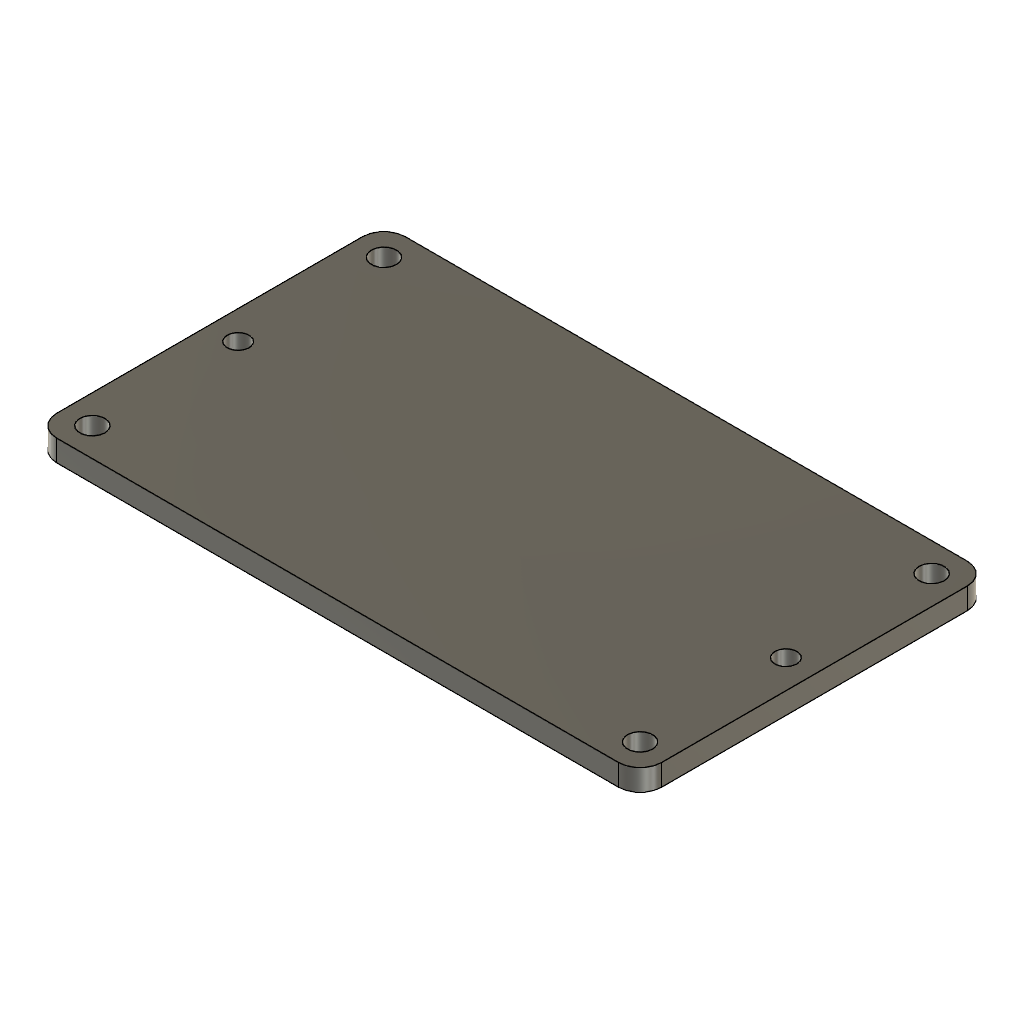
Hayai Bottom plate (Autodesk Fusion 360 design; units mm, degrees)
part number: 2026-09-20-15-42-52-633
Autodesk Fusion 360 part; units mm, degrees
sketch "Sketch1" plane through (0, 0, 0) normal (0, 0, 1) x (1, 0, 0)
  circle A0 centre (38.26, 20.3675) radius 1.75
  circle A1 centre (38.26, 0.0005) radius 1.525
  circle A2 centre (-38.26, -20.3675) radius 1.75
  circle A3 centre (-38.26, 20.3675) radius 1.75
  arc A4 (-39.26, 24.3675) -> (-42.26, 21.3675) centre (-39.26, 21.3675) ccw
  line L0 (-39.26, 24.3675) -> (39.26, 24.3675)
  line L1 (-42.26, -21.3675) -> (-42.26, 21.3675)
  circle A5 centre (-38.26, 0.0005) radius 1.525
  arc A6 (42.26, 21.3675) -> (39.26, 24.3675) centre (39.26, 21.3675) ccw
  line L2 (42.26, 21.3675) -> (42.26, -21.3675)
  arc A7 (-42.26, -21.3675) -> (-39.26, -24.3675) centre (-39.26, -21.3675) ccw
  line L3 (39.26, -24.3675) -> (-39.26, -24.3675)
  arc A8 (39.26, -24.3675) -> (42.26, -21.3675) centre (39.26, -21.3675) ccw
  circle A9 centre (38.26, -20.3675) radius 1.75
  point P0 (-42.26, -24.3675)
  dimension "d32" = 3.05
  dimension "d33" = 3.05
  dimension "d34" = 20.368
  dimension "d35" = 3
  dimension "d36" = 3
  dimension "d37" = 3
  dimension "d38" = 3
  dimension "d41" = 1.4142
  dimension "d42" = 4
  dimension "d45" = 4
  dimension "d51" = 20.368
  dimension "d52" = 48.735
  dimension "d55" = 4
  dimension "d56" = 4
  dimension "d59" = 3.5
  dimension "d62" = 84.52
  constraint horizontal L0
  constraint vertical L2
  constraint horizontal L3
  constraint vertical L1
  constraint tangent A4 L0
  constraint tangent A4 L1
  constraint tangent L0 A6
  constraint tangent A6 L2
  constraint tangent L2 A8
  constraint tangent L3 A8
  constraint tangent A7 L3
  constraint tangent L1 A7
  constraint equal A2 A3
  constraint equal A0 A9
  constraint equal A2 A9
  measures "d32" diameter of A5
  measures "d33" diameter of A1
  measures "d34" distance of A5.centre A2.centre
  measures "d35" radius of A4
  measures "d36" radius of A6
  measures "d37" radius of A8
  measures "d38" radius of A7
  measures "d41" distance of A8.centre A9.centre
  measures "d42" distance of L3 A9.centre
  measures "d45" distance of A3.centre L0
  measures "d51" distance of A1.centre A9.centre
  measures "d52" distance of L0 L3
  measures "d55" distance of A2.centre L3
  measures "d56" distance of A0.centre L0
  measures "d59" diameter of A2
  measures "d62" distance of L1 L2
extrude "Extrude8" add sketch "Sketch1" along normal blind 3
extrude "Extrude1" [suppressed]
extrude "Extrude2" [suppressed]
extrude "Extrude3" [suppressed]
extrude "Extrude4" [suppressed]
extrude "Extrude5" [suppressed]
extrude "Extrude6" [suppressed]
extrude "Extrude7" [suppressed]
equation "d41 = ( sqrt(2) ) * 1 mm"
